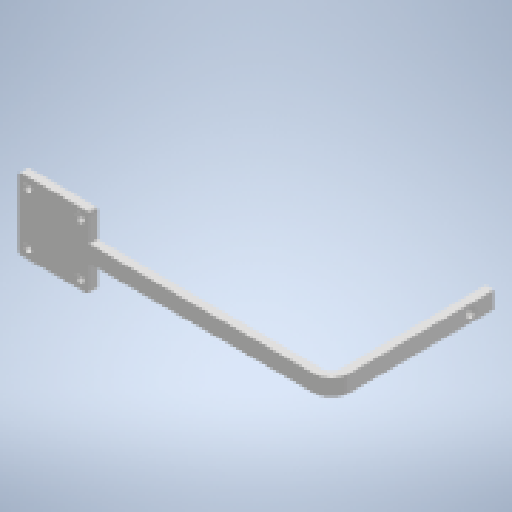
# Autodesk Inventor part: corredera
Saved by Autodesk Inventor 2023 (Build 270158000, 158)
## iProperties
Created: 2023-03-05
Part Number: corredera
Material: Generic
Document SubType Name: Sheet Metal
Designer: angel
Density: 1 g/cm^3
Sheet Metal Rule: Default_mm
Appearance: Default
Author: angel
Autodesk Inventor part; units mm, degrees
ref_plane "YZ Plane" through (0, 0, 0) normal (1, 0, 0) x (0, 1, 0)
ref_plane "XZ Plane" through (0, 0, 0) normal (0, 1, 0) x (-1, 0, 0)
ref_plane "XY Plane" through (0, 0, 0) normal (0, 0, 1) x (1, 0, 0)
sketch "Sketch1" plane through (0, 0, 0) normal (0, 0, 1) x (1, 0, 0)
  line L0 (-21.15, 19.15) -> (-21.15, -19.15)
  line L1 (21.15, -19.15) -> (21.15, 19.15)
  line L2 (19.15, 21.15) -> (-19.15, 21.15)
  line L3 (-19.15, -21.15) -> (19.15, -21.15)
  line L4 (159.3629, -5.0795) -> (159.3629, 4.9205)
  line L5 (159.3629, -5.0795) -> (159.3629, 4.9205)
  line L6 (159.3629, 4.9205) -> (138.2729, 4.9205)
  line L7 (138.2729, -5.0795) -> (159.3629, -5.0795)
  circle A0 centre (-15.5, -15.5) radius 2.55
  circle A1 centre (15.5, 15.5) radius 2.55
  circle A2 centre (-15.5, 15.5) radius 2.55
  circle A3 centre (15.5, -15.5) radius 2.55
  line L8 (-21.15, -19.15) -> (-21.15, 19.15)
  line L9 (-19.15, 21.15) -> (19.15, 21.15)
  line L10 (21.15, 19.15) -> (21.15, -19.15)
  line L11 (19.15, -21.15) -> (-19.15, -21.15)
  arc A4 (-21.15, -19.15) -> (-19.15, -21.15) centre (-19.15, -19.15) ccw
  arc A5 (-19.15, 21.15) -> (-21.15, 19.15) centre (-19.15, 19.15) ccw
  arc A6 (21.15, 19.15) -> (19.15, 21.15) centre (19.15, 19.15) ccw
  arc A7 (19.15, -21.15) -> (21.15, -19.15) centre (19.15, -19.15) ccw
  circle A8 centre (-15.5, -15.5) radius 2.55
  circle A9 centre (-15.5, 15.5) radius 2.55
  circle A10 centre (15.5, 15.5) radius 2.55
  circle A11 centre (15.5, -15.5) radius 2.55
  line L12 (159.3629, -5.0795) -> (21.15, -5.0795)
  line L13 (159.3629, -5.0795) -> (159.3629, 4.9205)
  line L14 (159.3629, 4.9205) -> (21.15, 4.9205)
  point P0 (0, 0)
  dimension "d0" = 2
  measures "d0" radius of A4
sketch "Sketch2" plane through (159.3629, -5.0795, 0) normal (1, 0, 0) x (0, 0, -1)
  line L0 (91.2, 0) -> (91.2, 10)
  line L1 (65, 0) -> (65, 10)
  circle A0 centre (78.1, 5) radius 2.75
  line L2 (-5, 10) -> (-5, 0)
  line L3 (0, 10) -> (-5, 10)
  line L4 (0, 0) -> (-5, 0)
  line L5 (-5, 10) -> (91.2, 10)
  line L6 (91.2, 10) -> (91.2, 0)
  line L7 (91.2, 0) -> (-5, 0)
  line L8 (-5, 0) -> (-5, 10)
  circle A1 centre (78.1, 5) radius 2.75
  point P0 (0, 5.0795)
extrude "Plate1" add sketch "Sketch1" along normal blind 5
sheet face with bend "Face2" sketch "Sketch2" thickness 5 toward (1, 0, 0) bend radius 5
bend "Bend1"
equation "\"d1\" = Thickness"
equation "\"d2\" = BendRadius"
equation "\"d3\" = BendReliefWidth"
equation "\"d5\" = MinimumRemnant"
equation "\"d4\" = BendReliefDepth"
equation "\"d6\" = TransitionRadius"
equation "\"BendRadius\" = Thickness"
equation "\"BendReliefWidth\" = Thickness"
equation "\"BendReliefDepth\" = 0.5 * Thickness"
equation "\"TransitionRadius\" = BendRadius"
equation "\"JacobiRadiusSize\" = BendRadius"
equation "\"GapSize\" = Thickness"
equation "\"Thickness\" = 5"
equation "\"MinimumRemnant\" = 10"
body "Solid1"
